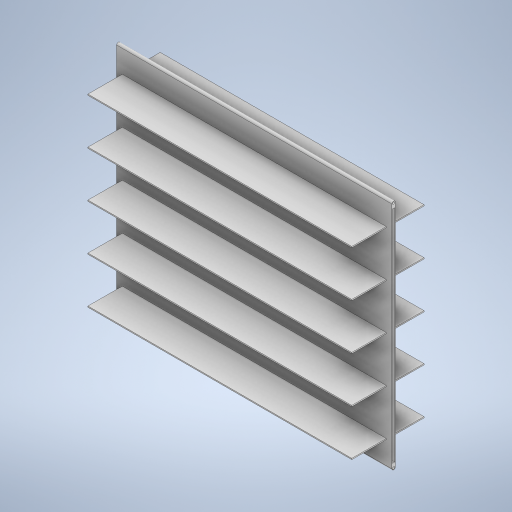
# Autodesk Inventor part: Layered Belt
Saved by Autodesk Inventor 2024 (Build 280153000, 153)
## iProperties
Created: 2024-09-18
Part Number: Layered Belt
Material: Generic
Document SubType Name: Modeling
Designer: srira
Density: 1 g/cm^3
Appearance: Default
Author: srira
Autodesk Inventor part; units mm, degrees
ref_plane "YZ Plane" through (0, 0, 0) normal (1, 0, 0) x (0, 1, 0)
ref_plane "XZ Plane" through (0, 0, 0) normal (0, 1, 0) x (-1, 0, 0)
ref_plane "XY Plane" through (0, 0, 0) normal (0, 0, 1) x (1, 0, 0)
sketch "Sketch1" plane through (0, 0, 0) normal (1, 0, 0) x (0, 1, 0)
  circle A0 centre (500, 0) radius 5
  arc A1 (500, -7.5) -> (500, 7.5) centre (500, 0) ccw
  circle A2 centre (-500, 0) radius 5
  arc A3 (-500, 7.5) -> (-500, -7.5) centre (-500, 0) ccw
  line L0 (500, -7.5) -> (-500, -7.5)
  line L1 (500, 7.5) -> (-500, 7.5)
  line L2 (-480, 5) -> (480, 5)
  line L3 (480, 5) -> (480, -5)
  line L4 (480, -5) -> (-480, -5)
  line L5 (-480, -5) -> (-480, 5)
  line L6 (-480, 5) -> (480, -5) construction
  line L7 (480, 5) -> (-480, -5) construction
  point P0 (0, 0)
  dimension "d0" = 10
  dimension "d1" = 15
  dimension "d2" = 10
  dimension "d3" = 15
  dimension "d4" = 1000
  dimension "d5" = 1000
  dimension "d6" = 960
  dimension "d7" = 10
  constraints: 16 end point, 4 centre point, 4 point on circle, 2 coincident, 2 midpoint, 2 parallel, 1 horizontal, 1 perpendicular
  measures "d0" diameter of A0
  measures "d1" diameter of A1
  measures "d2" diameter of A2
  measures "d3" diameter of A3
  measures "d4" distance of L0.start L0.end
  measures "d5" distance of L1.start L1.end
  measures "d6" distance of L3.end L4.end
  measures "d7" distance of L2.end L3.end
extrude "Extrusion1" add sketch "Sketch1" along normal blind 1200
sketch "Sketch2" plane through (0, -500, 7.5) normal (0, 0, 1) x (1, 0, 0)
  line L0 (25, 902.5) -> (1175, 902.5)
  line L1 (1175, 902.5) -> (1175, 897.5)
  line L2 (1175, 897.5) -> (25, 897.5)
  line L3 (25, 897.5) -> (25, 902.5)
  line L4 (25, 902.5) -> (1175, 897.5) construction
  line L5 (1175, 902.5) -> (25, 897.5) construction
  line L6 (1175, 697.5) -> (25, 697.5)
  line L7 (25, 702.5) -> (1175, 702.5)
  line L8 (25, 697.5) -> (25, 702.5)
  line L9 (1175, 702.5) -> (1175, 697.5)
  line L10 (1175, 497.5) -> (25, 497.5)
  line L11 (25, 502.5) -> (1175, 502.5)
  line L12 (25, 497.5) -> (25, 502.5)
  line L13 (1175, 502.5) -> (1175, 497.5)
  line L14 (1175, 297.5) -> (25, 297.5)
  line L15 (25, 302.5) -> (1175, 302.5)
  line L16 (25, 297.5) -> (25, 302.5)
  line L17 (1175, 302.5) -> (1175, 297.5)
  line L18 (1175, 97.5) -> (25, 97.5)
  line L19 (25, 102.5) -> (1175, 102.5)
  line L20 (25, 97.5) -> (25, 102.5)
  line L21 (1175, 102.5) -> (1175, 97.5)
  point P0 (600, 900)
  dimension "d10" = 1150
  dimension "d11" = 5
  dimension "d14" = 200
  constraints: 44 end point, 2 midpoint, 2 parallel, 1 collinear, 1 horizontal, 1 perpendicular, 1 vertical, 31 other
  measures "d10" distance of L1.end L2.end
  measures "d11" distance of L0.end L1.end
  measures "d14" distance of L1.end L6.start
extrude "Extrusion2" add sketch "Sketch2" along normal blind 150
sketch "Sketch3" plane through (0, -500, -7.5) normal (0, 0, -1) x (-1, 0, 0)
  line L0 (-25, 897.5) -> (-1175, 897.5) projected
  line L1 (-1175, 902.5) -> (-25, 902.5)
  line L2 (-25, 902.5) -> (-25, 897.5)
  line L3 (-25, 897.5) -> (-1175, 897.5)
  line L4 (-1175, 897.5) -> (-1175, 902.5)
  line L5 (-1175, 902.5) -> (-25, 897.5) construction
  line L6 (-25, 902.5) -> (-1175, 897.5) construction
  line L7 (-1175, 702.5) -> (-25, 702.5)
  line L8 (-25, 697.5) -> (-1175, 697.5)
  line L9 (-1175, 697.5) -> (-1175, 702.5)
  line L10 (-25, 702.5) -> (-25, 697.5)
  line L11 (-1175, 502.5) -> (-25, 502.5)
  line L12 (-25, 497.5) -> (-1175, 497.5)
  line L13 (-1175, 497.5) -> (-1175, 502.5)
  line L14 (-25, 502.5) -> (-25, 497.5)
  line L15 (-1175, 302.5) -> (-25, 302.5)
  line L16 (-25, 297.5) -> (-1175, 297.5)
  line L17 (-1175, 297.5) -> (-1175, 302.5)
  line L18 (-25, 302.5) -> (-25, 297.5)
  line L19 (-1175, 102.5) -> (-25, 102.5)
  line L20 (-25, 97.5) -> (-1175, 97.5)
  line L21 (-1175, 97.5) -> (-1175, 102.5)
  line L22 (-25, 102.5) -> (-25, 97.5)
  point P0 (0, 500)
  point P1 (-600, 900)
  dimension "d21" = 5
  dimension "d24" = 200
  constraints: 44 end point, 2 midpoint, 2 parallel, 1 collinear, 1 horizontal, 1 perpendicular, 1 vertical, 31 other
  measures "d21" distance of L1.end L0.start
  measures "d24" distance of L1.start L7.start
extrude "Extrusion3" add sketch "Sketch3" along normal blind 150
body "Solid1"
